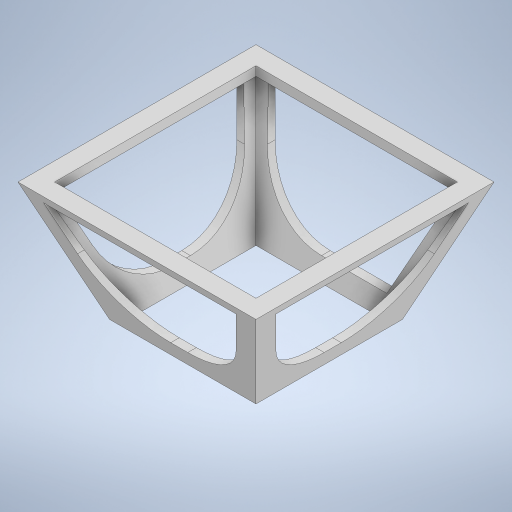
# Autodesk Inventor part: feet
Saved by Autodesk Inventor 2023 (Build 270158000, 158)
## iProperties
Created: 2023-05-03
Part Number: feet
Material: Generic
Document SubType Name: Modeling
Designer: ringl
Density: 1 g/cm^3
Appearance: Default
Author: ringl
Autodesk Inventor part; units mm, degrees
sketch "Sketch1" plane through (0, 0, 0) normal (0, 1, 0) x (-1, 0, 0)
  line L0 (0, 0) -> (80, 0)
  line L1 (80, 0) -> (80, -80)
  line L2 (80, -80) -> (0, -80)
  line L3 (0, -80) -> (0, 0)
  dimension "d0" = 80
  dimension "d1" = 80
  constraints: 8 end point, 2 parallel, 1 horizontal, 1 perpendicular
  measures "d0" distance of L1.end L2.end
  measures "d1" distance of L0.end L1.end
ref_plane "Work Plane1" through (0, 70, 0) normal (0, 1, 0) x (-1, 0, 0)
sketch "Sketch2" plane through (0, 70, 0) normal (0, 1, 0) x (-1, 0, 0)
  line L0 (100, 30) -> (-30, 30)
  line L1 (-30, 30) -> (-30, -100)
  line L2 (-30, -100) -> (100, -100)
  line L3 (100, -100) -> (100, 30)
  point P0 (0, 0)
  dimension "d9" = 30
  dimension "d10" = 130
  dimension "d13" = 130
  dimension "d15" = 30
  constraints: 8 end point, 2 parallel, 1 horizontal, 1 perpendicular
  measures "d9" distance from line of L0 point (0, 0)
  measures "d10" distance of L0.end L1.end
  measures "d13" distance of L0.start L0.end
  measures "d15" distance from line of L1 point (0, 0)
loft "Loft1" add profiles "Sketch2", "Sketch1"
sketch "Sketch3" plane through (-80, 0, 0) normal (0, -1, 0) x (1, 0, 0)
  line L0 (75, -5) -> (5, -5)
  line L1 (5, -5) -> (5, -75)
  line L2 (5, -75) -> (75, -75)
  line L3 (75, -75) -> (75, -5)
  line L4 (0, 0) -> (80, 0) projected
  line L5 (80, 0) -> (80, -80) projected
  line L6 (80, -80) -> (0, -80) projected
  line L7 (0, -80) -> (0, 0) projected
  dimension "d20" = 5
  dimension "d21" = 5
  dimension "d22" = 5
  dimension "d23" = 5
  constraints: 8 end point, 2 parallel, 1 horizontal, 1 perpendicular
  measures "d20" distance between parallel lines of L4 L0
  measures "d21" distance between parallel lines of L5 L3
  measures "d22" distance between parallel lines of L6 L2
  measures "d23" distance between parallel lines of L7 L1
ref_plane "Work Plane2" through (-100, 65, 30) normal (0, 1, 0) x (1, 0, 0)
sketch "Sketch4" plane through (-100, 65, 30) normal (0, 1, 0) x (1, 0, 0)
  line L0 (130, 0) -> (100, 30) projected
  line L1 (0, 130) -> (20, 110) projected
  line L2 (125, 5) -> (5, 5)
  line L3 (5, 5) -> (5, 125)
  line L4 (5, 125) -> (125, 125)
  line L5 (125, 125) -> (125, 5)
  line L6 (0, 0) -> (130, 0) projected
  line L7 (130, 130) -> (0, 130) projected
  dimension "d25" = 5
  dimension "d26" = 5
  constraints: 8 end point, 2 parallel, 2 point on line, 1 horizontal, 1 perpendicular
  measures "d25" distance between parallel lines of L6 L2
  measures "d26" distance between parallel lines of L7 L4
loft "Loft2" cut profiles "Sketch4", "Sketch3" contours all / L3 L2 L1 L0
ref_plane "Work Plane3" through (0, 0, 35.5) normal (0, 0, 1) x (1, 0, 0)
sketch "Sketch5" plane through (0, 0, 35.5) normal (0, 0, 1) x (1, 0, 0)
  line L0 (7.8637, 65) -> (-88.1713, 65)
  line L1 (-88.1713, 65) -> (-72.457, 10)
  line L2 (-72.457, 10) -> (-6.594, 10)
  line L3 (-6.594, 10) -> (16.9775, 65)
  line L4 (16.9775, 65) -> (7.8637, 65)
  line L5 (30, 70) -> (0, 0) projected
  line L6 (-100, 70) -> (30, 70) projected
  line L7 (-100, 70) -> (-80, 0) projected
  line L8 (-80, 0) -> (0, 0) projected
  dimension "d32" = 10
  dimension "d34" = 5
  dimension "d36" = 10
  dimension "d37" = 10
  constraints: 10 end point, 3 parallel, 1 collinear, 1 horizontal, 1 point on line
  measures "d32" distance from line of L5 L3.end
  measures "d34" distance between parallel lines of L6 L0
  measures "d36" distance between parallel lines of L7 L1
  measures "d37" distance between parallel lines of L8 L2
extrude "Extrusion1" cut sketch "Sketch5" against normal through all contours L4 L3 L2 L1 L0
ref_plane "Work Plane4" through (65, 0, 0) normal (1, 0, 0) x (0, 1, 0)
sketch "Sketch6" plane through (65, 0, 0) normal (1, 0, 0) x (0, 1, 0)
  line L0 (65, -88.1713) -> (10, -72.457)
  line L1 (10, -72.457) -> (10, -6.594)
  line L2 (10, -6.594) -> (65, 16.9775)
  line L3 (65, 16.9775) -> (65, -88.1713)
  line L4 (70, 30) -> (70, -100) projected
  line L5 (70, -100) -> (0, -80) projected
  line L6 (70, 30) -> (0, 0) projected
  line L7 (0, 0) -> (0, -80) projected
  dimension "d41" = 5
  dimension "d43" = 10
  dimension "d44" = 10
  dimension "d45" = 10
  constraints: 8 end point, 3 parallel, 1 vertical
  measures "d41" distance between parallel lines of L4 L3
  measures "d43" distance between parallel lines of L6 L2
  measures "d44" distance between parallel lines of L5 L0
  measures "d45" distance between parallel lines of L7 L1
extrude "Extrusion2" cut sketch "Sketch6" against normal through all contours L0 L1 L2 L3
fillet "Fillet1" radius 40 7 edges at (1.9505, 10, -72.457) (-72.457, 10, -80.467) (-80.467, 10, -72.457) (-80.467, 10, -6.594) (-6.594, 10, 1.9505) (1.9505, 10, -6.594) (-72.457, 10, 1.9505)
sketch "Sketch7" plane through (-100, 70, 30) normal (0, 1, 0) x (1, 0, 0)
  line L0 (10, 10) -> (120, 10)
  line L1 (120, 10) -> (120, 120)
  line L2 (120, 120) -> (10, 120)
  line L3 (10, 120) -> (10, 10)
  line L4 (130, 0) -> (130, 130) projected
  line L5 (0, 0) -> (130, 0) projected
  line L6 (130, 130) -> (0, 130) projected
  line L7 (0, 130) -> (0, 0) projected
  point P0 (100, 30)
  dimension "d49" = 10
  dimension "d50" = 10
  dimension "d51" = 10
  dimension "d52" = 10
  constraints: 8 end point, 2 parallel, 1 horizontal, 1 perpendicular
  measures "d49" distance between parallel lines of L4 L1
  measures "d50" distance between parallel lines of L5 L0
  measures "d51" distance between parallel lines of L6 L2
  measures "d52" distance between parallel lines of L7 L3
extrude "Extrusion3" cut sketch "Sketch7" against normal blind 10 contours L3 L2 L1 L0
body "Solid1"
